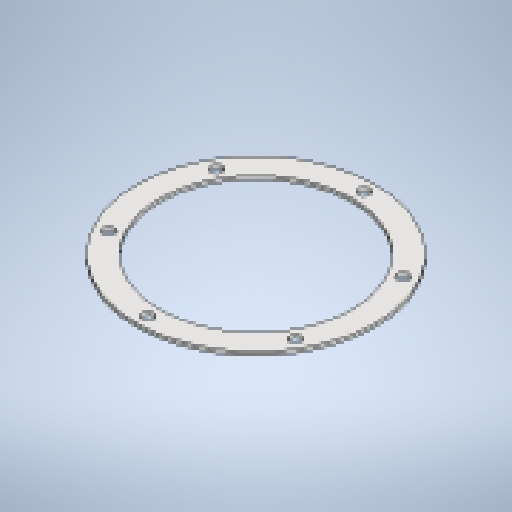
# Autodesk Inventor part: ДМФ 041 кольцо под шпильки КОРМА
Saved by Autodesk Inventor 2025.1 (Build 291241020, 241B)
## iProperties
Created: 2024-04-23
Part Number: ДМФ 041 кольцо под шпильки КОРМА
Material: Generic
Document SubType Name: Sheet Metal
Designer: admin
Density: 1 g/cm^3
Appearance: Default
Sheet Metal Rule: Default
Flat Pattern Width: 20.5 cm
Flat Pattern Length: 20.5 cm
Flat Pattern Area: 420.25 cm^2
Sheet Metal Width: 205.000 mm
Sheet Metal Length: 205.000 mm
Sheet Metal Area: 42025.000 mm^2
Stock Number: ДМФ 041 кольцо под шпильки КОРМА
back_steel_circle_диам_центров: 185.000 mm
back_steel_circle_ширина_кольца: 40,000 mm
back_steel_circle_диам_шпильки: 10,000 mm
back_steel_circle_кол_шпилек: 6,000 ul
back_steel_circle_внутр_диам: 165.000 mm
back_steel_circle_проходной_диаметр: 125.000 mm
Author: admin
Autodesk Inventor part; units mm, degrees
ref_plane "YZ Plane" through (0, 0, 0) normal (1, 0, 0) x (0, 1, 0)
ref_plane "XZ Plane" through (0, 0, 0) normal (0, 1, 0) x (-1, 0, 0)
ref_plane "XY Plane" through (0, 0, 0) normal (0, 0, 1) x (1, 0, 0)
sketch "Sketch1" plane through (0, 0, 0) normal (0, 0, 1) x (1, 0, 0)
  circle A0 centre (0, 0) radius 82.5
  circle A1 centre (0, 0) radius 102.5
  circle A2 centre (0, 0) radius 92.5 construction
  line L0 (0, 102.5) -> (0, 82.5) construction
  point P0 (0, 92.5)
  dimension "d30" = 165
  dimension "d32" = 205
extrude "Plate1" add sketch "Sketch1" along normal blind 3
sketch "Sketch2" plane through (0, 0, 3) normal (0, 0, 1) x (1, 0, 0)
  circle A0 centre (0, 0) radius 82.5 construction
  circle A1 centre (0, 0) radius 102.5 construction
  circle A2 centre (0, 0) radius 102.5 construction
  circle A3 centre (0, 0) radius 82.5 construction
  circle A4 centre (0, -92.5) radius 5
  circle A5 centre (0, 0) radius 92.5 construction
  dimension "d31" = 185
  dimension "d21" = 10
  constraints: 1 centre point, 1 coincident, 1 vertical alignment, 2 other
  measures "d21" diameter of A4
extrude "Extrusion1" cut sketch "Sketch2" against normal through all
pattern_circular "Circular Pattern2" count 6 over 360 about axis through (0, 0, 0) along (0, 0, 1) of "Extrusion1"
equation "\"d30\" = back_steel_circle_внутр_диам"
equation "\"d32\" = back_steel_circle_внутр_диам + back_steel_circle_ширина_кольца"
equation "\"d31\" = back_steel_circle_диам_центров"
equation "\"d21\" = back_steel_circle_диам_шпильки"
equation "\"d2\" = Thickness"
equation "\"BendRadius\" = Thickness"
equation "\"BendReliefWidth\" = Thickness"
equation "\"BendReliefDepth\" = 0.5 * Thickness"
equation "\"CornerReliefSize\" = 4 * Thickness"
equation "\"MinimumRemnant\" = 2 * Thickness"
equation "\"TransitionRadius\" = BendRadius"
equation "\"JacobiRadiusSize\" = BendRadius"
equation "\"GapSize\" = Thickness"
equation "\"back_steel_circle_диам_центров\" = back_steel_circle_внутр_диам + 0.5 * back_steel_circle_ширина_кольца"
equation "\"back_steel_circle_диам_шпильки\" = 10"
equation "\"back_steel_circle_проходной_диаметр\" = 125"
equation "\"back_steel_circle_внутр_диам\" = 165"
equation "\"back_steel_circle_ширина_кольца\" = 40"
equation "\"Thickness\" = 3"
body "Solid1"
